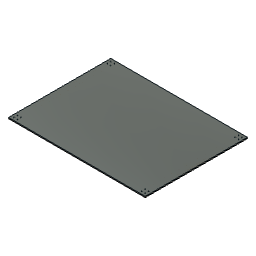
_base plate.83a4b455-5637-4f7c-b5de-213f8b637dbf (Autodesk Fusion 360 design; units mm, degrees)
Autodesk Fusion 360 part; units mm, degrees
sketch "Sketch1" plane through (0, 0, 0) normal (0, 0, 1) x (1, 0, 0)
  line L0 (0, 0) -> (793, 0)
  line L1 (793, 0) -> (793, 593)
  line L2 (793, 593) -> (0, 593)
  line L3 (0, 593) -> (0, 0)
  dimension "d1" = 793
  dimension "d2" = 593
  constraint horizontal L0
  constraint vertical L1
  constraint horizontal L2
  constraint vertical L3
  constraint coincident L0.start L3.end
  measures "d1" distance of L0.start L0.end
  measures "d2" distance of L0.start L2.end
extrude "Extrude1" add sketch "Sketch1" along normal blind 6
sketch "Sketch2" plane through (0, 0, 6) normal (0, 0, 1) x (-1, 0, 0)
  line L0 (0, -593) -> (0, 0)
  line L1 (0, 0) -> (-793, 0)
  line L2 (-793, 0) -> (-793, -593)
  line L3 (-793, -593) -> (0, -593)
  line L4 (0, 0) -> (-6, 0)
  line L5 (-6, 0) -> (-6, -6)
  line L6 (-6, -6) -> (0, -6)
  line L7 (0, -6) -> (0, 0)
  line L8 (-793, -593) -> (-787, -593)
  line L9 (-787, -593) -> (-787, -587)
  line L10 (-787, -587) -> (-793, -587)
  line L11 (-793, -587) -> (-793, -593)
  line L12 (-787, -587) -> (-6, -587)
  line L13 (-6, -587) -> (-6, -6)
  line L14 (-6, -6) -> (-787, -6)
  line L15 (-787, -6) -> (-787, -587)
  line L16 (-6, -6) -> (-36, -6)
  line L17 (-6, -36) -> (-6, -6)
  line L18 (-6, -6) -> (-16, -6)
  line L19 (-6, -16) -> (-6, -6)
  circle A0 centre (-16, -16) radius 2.5
  circle A1 centre (-36, -36) radius 2.5
  circle A2 centre (-16, -36) radius 2.5
  circle A3 centre (-36, -16) radius 2.5
  dimension "d5" = 6
  dimension "d6" = 6
  dimension "d7" = 6
  dimension "d8" = 6
  dimension "d9" = 30
  dimension "d10" = 30
  dimension "d11" = 10
  dimension "d12" = 10
  dimension "d13" = 5
  dimension "d14" = 5
  dimension "d15" = 5
  dimension "d16" = 5
  constraint horizontal L4
  constraint vertical L5
  constraint horizontal L6
  constraint vertical L7
  constraint coincident L0.end L1.start
  constraint horizontal L8
  constraint vertical L9
  constraint horizontal L10
  constraint vertical L11
  constraint coincident L2.end L3.start
  constraint horizontal L12
  constraint vertical L13
  constraint horizontal L14
  constraint vertical L15
  constraint horizontal L16
  constraint vertical L17
  constraint horizontal L18
  constraint vertical L19
  measures "d5" distance of L0.end L4.end
  measures "d6" distance of L0.end L6.end
  measures "d7" distance of L2.end L8.end
  measures "d8" distance of L2.end L10.end
  measures "d9" distance of L5.end L16.end
  measures "d10" distance of L5.end L17.start
  measures "d11" distance of L5.end L18.end
  measures "d12" distance of L5.end L19.start
  measures "d13" diameter of A0
  measures "d14" diameter of A1
  measures "d15" diameter of A2
  measures "d16" diameter of A3
extrude "Extrude2" cut sketch "Sketch2" against normal blind 6 contours A0 | A1 | A2 | A3
pattern_linear "R-Pattern1" count 1 spacing 0 along (0, 0, 1) count 2 spacing 741 along (1, 0, 0) of "Extrude2"
pattern_linear "R-Pattern2" count 1 spacing 0 along (1, 0, 0) count 2 spacing 541 along (0, 1, 0) of "Extrude2", "R-Pattern1"
sketch "Sketch4" plane through (0, 0, 6) normal (0, 0, 1) x (-1, 0, 0)
  circle A0 centre (-777, -577) radius 2.5
  circle A1 centre (-777, -557) radius 2.5
  circle A2 centre (-757, -577) radius 2.5
  circle A3 centre (-757, -557) radius 2.5
  circle A4 centre (-36, -577) radius 2.5
  circle A5 centre (-36, -557) radius 2.5
  circle A6 centre (-16, -577) radius 2.5
  circle A7 centre (-16, -557) radius 2.5
  circle A8 centre (-777, -36) radius 2.5
  circle A9 centre (-777, -16) radius 2.5
  circle A10 centre (-757, -36) radius 2.5
  circle A11 centre (-757, -16) radius 2.5
  circle A12 centre (-36, -36) radius 2.5
  circle A13 centre (-36, -16) radius 2.5
  circle A14 centre (-16, -36) radius 2.5
  circle A15 centre (-16, -16) radius 2.5
  line L0 (0, -593) -> (0, 0)
  line L1 (0, 0) -> (-793, 0)
  line L2 (-793, 0) -> (-793, -593)
  line L3 (-793, -593) -> (0, -593)
